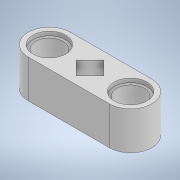
# Autodesk Inventor part: VexLegoBiggerCoupler
Saved by Autodesk Inventor 2020 (Build 240168000, 168)
## iProperties
Created: 2020-02-28
Part Number: VexLegoBiggerCoupler
Material: Generic
Document SubType Name: Modeling
Designer: Luke
Density: 1 g/cm^3
Appearance: Default
Author: Luke
Autodesk Inventor part; units mm, degrees
ref_plane "YZ Plane" through (0, 0, 0) normal (1, 0, 0) x (0, 1, 0)
ref_plane "XZ Plane" through (0, 0, 0) normal (0, 1, 0) x (-1, 0, 0)
ref_plane "XY Plane" through (0, 0, 0) normal (0, 0, 1) x (1, 0, 0)
sketch "Sketch1" plane through (0, 0, 0) normal (0, 1, 0) x (-1, 0, 0)
  line L0 (-8.001, 0) -> (8.001, 0) construction
  line L1 (-8.001, -4.191) -> (8.001, -4.191)
  line L2 (8.001, 4.191) -> (-8.001, 4.191)
  arc A0 (-8.001, 4.191) -> (-8.001, -4.191) centre (-8.001, 0) ccw
  arc A1 (8.001, -4.191) -> (8.001, 4.191) centre (8.001, 0) ccw
  line L3 (-2.6941, 0) -> (0, 2.6941)
  line L4 (0, 2.6941) -> (2.6941, 0)
  line L5 (2.6941, 0) -> (0, -2.6941)
  line L6 (0, -2.6941) -> (-2.6941, 0)
  line L7 (-2.6941, 0) -> (2.6941, 0) construction
  line L8 (0, 2.6941) -> (0, -2.6941) construction
  point P0 (0, 0)
  dimension "d0" = 8.001
  dimension "d1" = 8.382
  dimension "d2" = 3.81
  dimension "d3" = 3.81
  constraints: 20 end point, 4 point on circle, 4 tangent, 3 midpoint, 3 parallel, 2 centre point, 1 horizontal, 1 perpendicular
  measures "d0" distance of point (0, 0) L0.end
  measures "d1" diameter of A1
  measures "d2" distance of L4.end L5.end
  measures "d3" distance of L3.end L4.end
extrude "Extrusion1" add sketch "Sketch1" along normal blind 7.493
sketch "Sketch2" plane through (0, 7.493, 0) normal (0, 1, 0) x (1, 0, 0)
  circle A0 centre (-8.001, 0) radius 3.2385
  point P0 (0, 0)
  dimension "d6" = 8.001
  dimension "d7" = 6.477
  constraints: 1 centre point, 1 coincident
  measures "d6" distance of point (0, 0) point (-8.001, 0)
  measures "d7" diameter of A0
extrude "Extrusion2" cut sketch "Sketch2" against normal blind 0.7874
sketch "Sketch3" plane through (0, 7.493, 0) normal (0, 1, 0) x (1, 0, 0)
  circle A0 centre (8.001, 0) radius 3.2385
  point P0 (0, 0)
  dimension "d10" = 8.001
  dimension "d11" = 6.477
  constraints: 1 centre point, 1 coincident
  measures "d10" distance of point (0, 0) point (8.001, 0)
  measures "d11" diameter of A0
extrude "Extrusion3" cut sketch "Sketch3" against normal blind 0.7874
sketch "Sketch4" plane through (0, 0, 0) normal (0, -1, 0) x (1, 0, 0)
  circle A0 centre (8.001, 0) radius 3.2385 projected
  circle A1 centre (8.001, 0) radius 2.8575
  point P0 (0, 0)
  constraints: 1 centre point, 1 coincident
extrude "Extrusion4" cut sketch "Sketch4" against normal blind 0.7874 contours A0 | A1
sketch "Sketch5" plane through (0, 0, 0) normal (0, -1, 0) x (1, 0, 0)
  circle A0 centre (-8.001, 0) radius 3.2385 projected
  circle A1 centre (-8.001, 0) radius 2.8575
  point P0 (0, 0)
  constraints: 1 centre point, 1 coincident
extrude "Extrusion5" cut sketch "Sketch5" against normal blind 0.7874 contours A0 | A1
sketch "Sketch6" plane through (-8.001, 6.7056, 0) normal (0, 1, 0) x (1, 0, 0)
  circle A0 centre (0, 0) radius 2.7051
  point P0 (8.001, 0)
  dimension "d18" = 5.4102
  constraints: 1 centre point
  measures "d18" diameter of A0
extrude "Extrusion6" cut sketch "Sketch6" against normal through all
sketch "Sketch7" plane through (8.001, 6.7056, 0) normal (0, 1, 0) x (1, 0, 0)
  circle A0 centre (0, 0) radius 2.7051
  point P0 (-8.001, 0)
  dimension "d21" = 5.4102
  constraints: 1 centre point
  measures "d21" diameter of A0
extrude "Extrusion7" cut sketch "Sketch7" against normal through all
body "Solid1"
